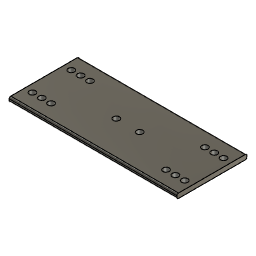
Attachment_top_short_new v2 (Autodesk Fusion 360 design; units mm, degrees)
Autodesk Fusion 360 part; units mm, degrees
sketch "Sketch7" plane through (0, 0, 0) normal (0, 0, 1) x (1, 0, 0)
  line L0 (0, 0) -> (108, 0)
  line L1 (0, 0) -> (0, 45)
  line L2 (0, 45) -> (108, 45)
  line L3 (108, 45) -> (108, 0)
  dimension "d135" = 108
  dimension "d136" = 45
  constraint coincident L0.start L1.start
  constraint horizontal L0
  constraint perpendicular L0 L1
  constraint perpendicular L1 L2
  constraint perpendicular L0 L3
  measures "d135" distance of L0.start L0.end
  measures "d136" distance of L0.start L1.end
extrude "Extrude7" add sketch "Sketch7" along normal blind 3
sketch "Sketch8" plane through (0, 0, 3) normal (0, 0, 1) x (-1, 0, 0)
  line L0 (0, 0) -> (-108, 0)
  line L1 (-108, 0) -> (-108, -45)
  line L2 (-108, -45) -> (0, -45)
  line L3 (0, -45) -> (0, 0)
  circle A0 centre (-5, -35) radius 2
  circle A1 centre (-5, -10) radius 2
  circle A2 centre (-11, -35) radius 2
  circle A3 centre (-17, -35) radius 2
  circle A4 centre (-11, -10) radius 2
  circle A5 centre (-17, -10) radius 2
  circle A6 centre (-46.5, -22.5) radius 2
  circle A7 centre (-103, -35) radius 2
  circle A8 centre (-103, -10) radius 2
  circle A9 centre (-97, -10) radius 2
  circle A10 centre (-91, -10) radius 2
  circle A11 centre (-91, -35) radius 2
  circle A12 centre (-97, -35) radius 2
  circle A13 centre (-61.5, -22.5) radius 2
  dimension "d142" = 6
  dimension "d143" = 6
  dimension "d144" = 6
  dimension "d145" = 6
  dimension "d146" = 4
  dimension "d147" = 4
  dimension "d148" = 4
  dimension "d149" = 4
  dimension "d150" = 4
  dimension "d151" = 4
  dimension "d153" = 4
  measures "d142" distance of A0.centre A2.centre
  measures "d143" distance of A2.centre A3.centre
  measures "d144" distance of A1.centre A4.centre
  measures "d145" distance of A4.centre A5.centre
  measures "d146" diameter of A0
  measures "d147" diameter of A1
  measures "d148" diameter of A2
  measures "d149" diameter of A3
  measures "d150" diameter of A4
  measures "d151" diameter of A5
  measures "d153" diameter of A6
extrude "Extrude8" cut sketch "Sketch8" against normal blind 3 contours A0 | A1 | A2 | A3 | A4 | A5 | A6 | A7 | A8 | A9 | A10 | A11 | A12 | A13
fillet "Fillet13" radius 1 1 edges at (54, 0, 3)
fillet "Fillet14" radius 1 1 edges at (54, 0, 0)
fillet "Fillet15" radius 1 1 edges at (54, 45, 3)
fillet "Fillet16" radius 1 1 edges at (54, 45, 0)
